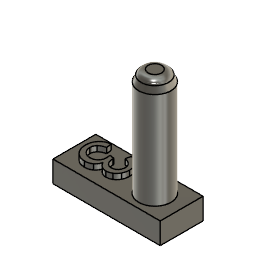
Pole3mm_v1 (Autodesk Fusion 360 design; units mm, degrees)
Autodesk Fusion 360 part; units mm, degrees
sketch "Sketch1" plane through (0, 0, 0) normal (0, 0, 1) x (1, 0, 0)
  line L0 (5, -2) -> (-5, -2)
  line L1 (-5, -2) -> (-5, 2)
  line L2 (-5, 2) -> (5, 2)
  line L3 (5, 2) -> (5, -2)
  line L4 (5, -2) -> (-5, 2) construction
  line L5 (-5, -2) -> (5, 2) construction
  line L6 (-2.0416, 1.4237) -> (-2.0416, -1.5763) construction
  line L7 (-2.0416, -1.5763) -> (-0.0416, -1.5763) construction
  line L8 (-0.0416, -1.5763) -> (-0.0416, 1.4237) construction
  line L9 (-0.0416, 1.4237) -> (-2.0416, 1.4237) construction
  circle A0 centre (2.5, 0) radius 1.5
  dimension "d2" = 4
  dimension "d3" = 0
  dimension "d4" = 3
  text T0 "3" font "Arial" height 4 align left top in box 3 x 2 at (-2.0416, 1.4237) x (0, -1) y (1, 0) spacing 1.01 kerned
  constraint horizontal L0
  constraint perpendicular L0 L1
  constraint parallel L0 L2
  constraint parallel L1 L3
  constraint coincident L4 origin
  constraint coincident L5 origin
  measures "d4" diameter of A0
extrude "Extrude1" add sketch "Sketch1" against normal blind 2 makes body 1
extrude "Extrude2" add sketch "Sketch1" along normal blind 0.5 text T0 bodies 1
extrude "Extrude3" add sketch "Sketch1" along normal blind 10 separate body contours A0 makes body 2
extrude "Extrude4" add sketch "Sketch1" against normal blind 2 contours A0 bodies 1 2
chamfer "Chamfer1" distance 0.4 distance2 1 1 edges at (1.1015, -0.5424, 10) measured on face at (2.9505, -0.3464, 10) tangent chain off on bodies 1
fillet "Fillet1" radius 0.7 1 edges at (1.4744, 0.3978, 10) on bodies 1
equation "d3 = '3'"
